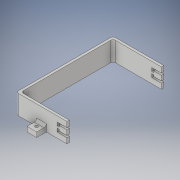
# Autodesk Inventor part: batery holder side opening
Saved by Autodesk Inventor 2019 (Build 230136000, 136)
## iProperties
Created: 2019-11-19
Part Number: batery holder side opening
Material: Generic
Document SubType Name: Modeling
Designer: User
Density: 1 g/cm^3
Appearance: Default
Author: User
Autodesk Inventor part; units mm, degrees
ref_plane "YZ Plane" through (0, 0, 0) normal (1, 0, 0) x (0, 1, 0)
ref_plane "XZ Plane" through (0, 0, 0) normal (0, 1, 0) x (-1, 0, 0)
ref_plane "XY Plane" through (0, 0, 0) normal (0, 0, 1) x (1, 0, 0)
sketch "Sketch1" plane through (0, 0, 0) normal (0, 1, 0) x (-1, 0, 0)
  line L0 (0, 0) -> (63.5, 0)
  line L1 (63.5, 0) -> (63.5, -3.175)
  line L2 (63.5, -3.175) -> (0, -3.175)
  line L3 (0, -3.175) -> (0, 0)
  line L4 (63.5, 0) -> (66.675, 0)
  line L5 (66.675, 0) -> (66.675, -127)
  line L6 (66.675, -127) -> (63.5, -127)
  line L7 (63.5, -127) -> (63.5, 0)
  line L8 (66.675, -127) -> (0, -127)
  line L9 (0, -127) -> (0, -123.825)
  line L10 (0, -123.825) -> (66.675, -123.825)
  line L11 (66.675, -123.825) -> (66.675, -127)
  dimension "d0" = 3.175
  dimension "d1" = 3.175
  dimension "d2" = 3.175
  dimension "d3" = 120.65
  dimension "d4" = 63.5
  constraints: 24 end point, 6 parallel, 3 horizontal, 3 perpendicular, 1 point on line
  measures "d0" distance between parallel lines of L0 L2
  measures "d1" distance of L8.end L9.end
  measures "d2" distance of L5.end L6.end
  measures "d3" distance between parallel lines of L10 L2
  measures "d4" distance between parallel lines of L9 L7
extrude "Extrusion1" add sketch "Sketch1" along normal blind 25.4
sketch "Sketch2" plane through (-66.675, 0, 0) normal (0, 0, 1) x (1, 0, 0)
  line L0 (66.675, 0) -> (66.675, 25.4) projected
  line L1 (66.675, 18.415) -> (53.975, 18.415)
  line L2 (53.975, 18.415) -> (53.975, 13.97)
  line L3 (56.515, 13.97) -> (56.515, 15.875)
  line L4 (56.515, 15.875) -> (66.675, 15.875)
  line L5 (53.975, 11.43) -> (53.975, 6.985)
  line L6 (53.975, 6.985) -> (66.675, 6.985)
  line L7 (105.3402, 6.985) -> (66.675, 6.985)
  line L8 (56.515, 9.525) -> (66.675, 9.525)
  line L9 (56.515, 9.525) -> (56.515, 11.43)
  line L10 (56.515, 13.97) -> (53.975, 13.97)
  line L11 (53.975, 11.43) -> (56.515, 11.43)
  line L12 (0, 0) -> (66.675, 0) projected
  dimension "d9" = 2.54
  dimension "d10" = 2.54
  dimension "d11" = 6.35
  dimension "d12" = 2.54
  dimension "d13" = 1.905
  dimension "d14" = 11.43
  dimension "d15" = 25.4
  dimension "d16" = 6.985
  dimension "d17" = 2.54
  dimension "d18" = 2.54
  dimension "d19" = 12.7
  dimension "d20" = 12.7
  constraints: 22 end point, 5 perpendicular, 4 point on line, 2 vertical, 1 horizontal
  measures "d9" distance between parallel lines of L1 L4
  measures "d10" distance between parallel lines of L8 L7
  measures "d11" distance between parallel lines of L4 L8
  measures "d12" distance between parallel lines of L10 L11
  measures "d13" distance between parallel lines of L8 L11
  measures "d14" distance between parallel lines of L1 L6
  measures "d15" distance of L0.start L0.end
  measures "d16" distance between parallel lines of L12 L6
  measures "d17" distance between parallel lines of L2 L3
  measures "d18" distance between parallel lines of L5 L9
  measures "d19" distance between parallel lines of L0 L2
  measures "d20" distance between parallel lines of L0 L5
extrude "Extrusion3" cut sketch "Sketch2" against normal through all
sketch "Sketch3" plane through (0, 0, 0) normal (0, -1, 0) x (1, 0, 0)
  line L0 (-26.9875, 0) -> (-39.6875, 0)
  line L1 (-39.6875, 0) -> (-39.6875, 12.7)
  line L2 (-39.6875, 12.7) -> (-26.9875, 12.7)
  line L3 (-26.9875, 12.7) -> (-26.9875, 0)
  line L4 (-66.675, 0) -> (0, 0) projected
  line L5 (-66.675, -127) -> (-66.675, 0) projected
  dimension "d26" = 12.7
  dimension "d27" = 12.7
  dimension "d28" = 66.675
  dimension "d29" = 26.9875
  dimension "d30" = 0
  constraints: 8 end point, 2 parallel, 1 horizontal, 1 perpendicular
  measures "d26" distance between parallel lines of L1 L3
  measures "d27" distance between parallel lines of L2 L0
  measures "d28" distance of L4.start L4.end
  measures "d29" distance between parallel lines of L5 L1
  measures "d30" distance between parallel lines of L4 L0
extrude "Extrusion4" add sketch "Sketch3" against normal blind 6.35
sketch "Sketch4" plane through (0, 6.35, 0) normal (0, 1, 0) x (1, 0, 0)
  line L0 (-26.9875, -12.7) -> (-26.9875, 0) projected
  line L1 (-39.6875, 0) -> (-26.9875, 0) projected
  line L2 (-39.6875, 0) -> (-39.6875, -12.7) projected
  line L3 (-39.6875, -12.7) -> (-26.9875, -12.7) projected
  point P0 (0, 0)
  point P1 (-33.3505, -6.4321)
hole "Hole1" at (-33.3505, 6.35, 6.4321) direction (0, -1, 0) diameter 3.81 end through all
ref_plane "Work Plane1" through (-66.675, 25.4, -63.5) normal (0, 0, 1) x (1, 0, 0)
mirror "Mirror1" about plane through (-66.675, 25.4, -63.5) normal (0, 0, 1) of "Extrusion4", "Hole1"
fillet "Fillet1" radius 3.175 2 edges at (-33.3375, 6.35, 0) (-33.3375, 6.35, -127)
fillet "Fillet2" radius 3.175 4 edges at (-66.675, 12.7, 0) (-66.675, 12.7, -127) (-63.5, 12.7, -123.825) (-63.5, 12.7, -3.175)
equation "\"d0\" = d2"
equation "\"d2\" = d1"
equation "\"d10\" = d9"
equation "\"d13\" = -0.5 * d12 + 0.5 * d11"
equation "\"d16\" = -0.5 * d14 + 0.5 * d15"
equation "\"d17\" = d9"
equation "\"d18\" = d17"
equation "\"d20\" = d19"
equation "\"d29\" = -0.5 * d26 + 0.5 * d28"
body "Solid1"
